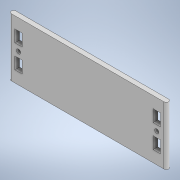
# Autodesk Inventor part: menteB
Saved by Autodesk Inventor 2020.2 (Build 242310000, 310)
## iProperties
Created: 2020-03-04
Part Number: menteB
Material: 一般
Document SubType Name: Modeling
Designer: touhu_zn72wdq
Density: 1 g/cm^3
Appearance: 既定
Author: touhu_zn72wdq
Autodesk Inventor part; units mm, degrees
ref_plane "YZ Plane" through (0, 0, 0) normal (1, 0, 0) x (0, 1, 0)
ref_plane "XZ Plane" through (0, 0, 0) normal (0, 1, 0) x (-1, 0, 0)
ref_plane "XY Plane" through (0, 0, 0) normal (0, 0, 1) x (1, 0, 0)
sketch "スケッチ1" plane through (0, 0, 0) normal (0, 0, 1) x (1, 0, 0)
  line L0 (0, 0) -> (135, 0)
  line L1 (135, 0) -> (135, 50)
  line L2 (135, 50) -> (0, 50)
  line L3 (0, 50) -> (0, 0)
  dimension "d0" = 135
  dimension "d1" = 50
  constraints: 8 end point, 2 parallel, 1 horizontal, 1 perpendicular
  measures "d0" distance of L2.end L1.end
  measures "d1" distance of L1.end L0.end
extrude "押し出し1" add sketch "スケッチ1" along normal blind 4
sketch "スケッチ2" plane through (0, 0, 4) normal (0, 0, 1) x (1, 0, 0)
  line L0 (5, 40.2) -> (11.3, 40.2)
  line L1 (11.3, 40.2) -> (11.3, 29.9)
  line L2 (11.3, 29.9) -> (5, 29.9)
  line L3 (5, 29.9) -> (5, 40.2)
  line L4 (135, 50) -> (0, 50) projected
  line L5 (0, 50) -> (0, 0) projected
  line L6 (0, 25) -> (135, 25)
  line L7 (135, 0) -> (135, 50) projected
  line L8 (67.5, 50) -> (67.5, 0)
  line L9 (0, 0) -> (135, 0) projected
  line L10 (5, 9.8) -> (11.3, 9.8)
  line L11 (11.3, 9.8) -> (11.3, 20.1)
  line L12 (11.3, 20.1) -> (5, 20.1)
  line L13 (5, 20.1) -> (5, 9.8)
  line L14 (130, 40.2) -> (123.7, 40.2)
  line L15 (123.7, 40.2) -> (123.7, 29.9)
  line L16 (123.7, 29.9) -> (130, 29.9)
  line L17 (130, 29.9) -> (130, 40.2)
  line L18 (135, 25) -> (0, 25)
  line L19 (130, 9.8) -> (123.7, 9.8)
  line L20 (123.7, 9.8) -> (123.7, 20.1)
  line L21 (123.7, 20.1) -> (130, 20.1)
  line L22 (130, 20.1) -> (130, 9.8)
  dimension "d4" = 6.3
  dimension "d5" = 10.3
  dimension "d6" = 9.8
  dimension "d7" = 5
  constraints: 38 end point, 14 symmetric about line, 4 midpoint, 2 parallel, 1 horizontal, 1 perpendicular
  measures "d4" distance of L1.end L2.end
  measures "d5" distance of L0.end L1.end
  measures "d6" distance between parallel lines of L4 L0
  measures "d7" distance between parallel lines of L5 L3
extrude "押し出し2" cut sketch "スケッチ2" against normal blind 10 contours L0 L1 L2 L3 | L13 L12 L11 L10 | L17 L16 L15 L14 | L19 L20 L21 L22
sketch "スケッチ3" plane through (0, 0, 4) normal (0, 0, 1) x (1, 0, 0)
  line L0 (11.3, 29.9) -> (5, 29.9) projected
  line L1 (0, 50) -> (0, 0) projected
  line L2 (135, 50) -> (0, 50) projected
  line L3 (67.5, 50) -> (67.5, 0)
  line L4 (0, 0) -> (135, 0) projected
  point P0 (8.15, 25)
  point P1 (126.85, 25)
  dimension "d10" = 4.9
  dimension "d11" = 8.15
  constraints: 2 end point, 2 midpoint, 1 symmetric about line
  measures "d10" distance from line of L0 point (8.15, 25)
  measures "d11" distance from line of L1 point (8.15, 25)
hole "穴1" at (8.15, 25, 4) at (126.85, 25, 4) direction (0, 0, -1) diameter 3.6 depth 4.5
fillet "フィレット1" radius 2 4 edges at (0, 25, 4) (0, 25, 0) (135, 25, 4) (135, 25, 0)
